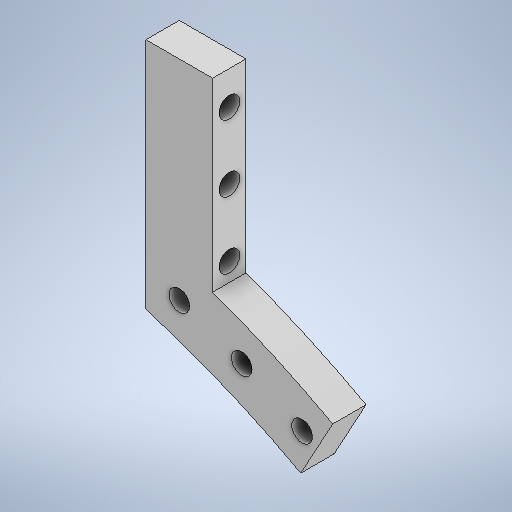
# Autodesk Inventor part: ring_to_plate
Saved by Autodesk Inventor 2025.1 (Build 291241000, 241)
## iProperties
Created: 2025-05-01
Part Number: ring_to_plate
Material: 一般
Document SubType Name: Modeling
Designer: yuki0520
Density: 1 g/cm^3
Appearance: 既定
Author: yuki0520
Autodesk Inventor part; units mm, degrees
ref_plane "YZ Plane" through (0, 0, 0) normal (1, 0, 0) x (0, 1, 0)
ref_plane "XZ Plane" through (0, 0, 0) normal (0, 1, 0) x (-1, 0, 0)
ref_plane "XY Plane" through (0, 0, 0) normal (0, 0, 1) x (1, 0, 0)
derived "zzz_sekkei.ipt"
sketch "スケッチ1" plane through (0, 0, 0) normal (0, 0, 1) x (1, 0, 0)
  circle A0 centre (0, 0) radius 120
  line L0 (12.25, -196) -> (-12.25, -196)
  line L1 (-12.25, -196) -> (-12.25, -120)
  line L2 (-12.25, -120) -> (12.25, -120)
  line L3 (12.25, -120) -> (12.25, -196)
  line L4 (12.25, -196) -> (-12.25, -120) construction
  line L5 (-12.25, -196) -> (12.25, -120) construction
  circle A1 centre (0, 0) radius 130
  line L6 (0, 130) -> (0, -130)
  line L7 (41.25, -164) -> (-95.75, -164)
  line L8 (-95.75, -164) -> (-95.75, -152)
  line L9 (-95.75, -152) -> (41.25, -152)
  line L10 (41.25, -152) -> (41.25, -164)
  line L11 (41.25, -164) -> (-95.75, -152) construction
  line L12 (-95.75, -164) -> (41.25, -152) construction
  line L13 (-12.25, -158) -> (12.25, -158)
  line L14 (34.25, -120) -> (34.25, -320)
  line L15 (34.25, -115.0084) -> (44.25, -115.0084)
  line L16 (44.25, -115.0084) -> (44.25, -150.0084)
  line L17 (44.25, -150.0084) -> (34.25, -150.0084)
  line L18 (34.25, -150.0084) -> (34.25, -115.0084)
  line L19 (34.25, -120) -> (44.25, -120)
  line L20 (0, 0) -> (62.2468, -114.1286)
  line L21 (0, 0) -> (37.1042, -124.5925)
  line L22 (30.3, 120) -> (-30.3, 120)
  line L23 (-30.3, 120) -> (-30.3, 138.5)
  line L24 (-30.3, 138.5) -> (30.3, 138.5)
  line L25 (30.3, 138.5) -> (30.3, 120)
  line L26 (30.3, 120) -> (-30.3, 138.5) construction
  line L27 (-30.3, 120) -> (30.3, 138.5) construction
  line L28 (34.25, 180) -> (34.25, 120)
  line L29 (34.25, 120) -> (70, 120)
  line L30 (34.25, 115.0084) -> (44.25, 115.0084)
  line L31 (44.25, 115.0084) -> (44.25, 150.0084)
  line L32 (44.25, 150.0084) -> (34.25, 150.0084)
  line L33 (34.25, 150.0084) -> (34.25, 115.0084)
  line L34 (0, 0) -> (37.1042, 124.5925)
  line L35 (0, 0) -> (62.2468, 114.1286)
  circle A2 centre (0, 0) radius 125
  point P0 (0, -158)
  point P1 (-27.25, -158)
  point P2 (0, 129.25)
  point P3 (34.25, 150.0084)
  point P4 (57.4586, 105.3495)
  point P5 (44.25, 122.2372)
  point P6 (39.25, 118.6779)
  point P7 (39.25, -118.6779)
  point P8 (34.25, -132.5084)
extrude "押し出し1" add sketch "スケッチ1" along normal blind 5 contours A0 L30 L31 A2 L35 | L34 A2 L31 L30 | L33 L29 A2 L34 | A2 L31 L29 A1 L35 | L28 A2 L29 | A2 L29 L34 | L34 L29 L31 A2 | L28 A1 L34 L29 A2 | L34 A1 L31 L29 | L29 L31 A1 | L28 L32 L31 A1
sketch "スケッチ2" plane through (34.25, 115.0084, 0) normal (-1, 0, 0) x (0, 0, 1)
  line L0 (0, 35) -> (0, 0) projected
  line L1 (0, 0) -> (5, 0) projected
  line L2 (5, 35) -> (5, 0) projected
  line L3 (0, 35) -> (5, 35) projected
  line L4 (2.5, 35) -> (2.5, 0)
  point P0 (0, -115.0084)
  point P1 (2.5, 30)
  point P2 (2.5, 20)
  point P3 (2.5, 10)
  dimension "d3" = 5
  dimension "d4" = 10
  dimension "d5" = 10
  constraints: 3 point on line, 2 end point, 2 midpoint
  measures "d3" distance from line of L3 point (2.5, 30)
  measures "d4" distance of point (2.5, 20) point (2.5, 30)
  measures "d5" distance of point (2.5, 10) point (2.5, 20)
hole "穴1" at (34.25, 145.0084, 2.5) at (34.25, 135.0084, 2.5) at (34.25, 125.0084, 2.5) direction (1, 0, 0) diameter 3.1 end through all
sketch "スケッチ3" plane through (34.25, 150.0084, 5) normal (0, 0, 1) x (1, 0, 0)
  circle A0 centre (-34.25, -150.0084) radius 120 projected
  circle A1 centre (-34.25, -150.0084) radius 125
  line L0 (0, 0) -> (0, -35) projected
  arc A2 (23.2086, -44.6589) -> (0, -35) centre (-34.25, -150.0084) ccw projected
  line L1 (23.2086, -44.6589) -> (27.9968, -35.8798) projected
  arc A3 (27.9968, -35.8798) -> (10, -27.7712) centre (-34.25, -150.0084) ccw projected
  line L2 (10, -27.7712) -> (10, 0) projected
  line L3 (10, 0) -> (0, 0) projected
  point P0 (23.411, -39.1021)
  point P1 (14.361, -34.8478)
  point P2 (5, -31.3306)
  dimension "d13" = 5
  dimension "d14" = 10
  dimension "d15" = 10
  dimension "d16" = 5
  constraints: 3 point on circle, 1 centre point
  measures "d13" radial gap between concentric circles of A0 A1
  measures "d14" distance of A1.end point (5, -31.331)
  measures "d15" distance of A1.start A1.end
  measures "d16" distance from line of L0 point (5, -31.331)
hole "穴2" at (57.661, 110.9063, 5) at (48.611, 115.1606, 5) at (39.25, 118.6779, 5) direction (0, 0, -1) diameter 3.1 end through all
